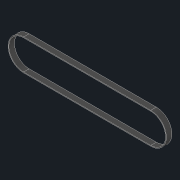
# Autodesk Inventor part: belt4
Saved by Autodesk Inventor 2021 (Build 250183000, 183)
## iProperties
Created: 2021-08-06
Part Number: belt4
Material: ゴム
Document SubType Name: Modeling
Designer: yuta0
Density: 0.93 g/cm^3
Appearance: ゴム - 黒
Author: yuta0
Autodesk Inventor part; units mm, degrees
ref_plane "YZ Plane" through (0, 0, 0) normal (1, 0, 0) x (0, 1, 0)
ref_plane "XZ Plane" through (0, 0, 0) normal (0, 1, 0) x (-1, 0, 0)
ref_plane "XY Plane" through (0, 0, 0) normal (0, 0, 1) x (1, 0, 0)
sketch "スケッチ1" plane through (0, 0, 0) normal (0, 0, 1) x (1, 0, 0)
  line L0 (-68, 0) -> (68, 0) construction
  line L1 (-68, -16.2338) -> (68, -16.2338)
  line L2 (68, 16.2338) -> (-68, 16.2338)
  arc A0 (-68, 16.2338) -> (-68, -16.2338) centre (-68, 0) ccw
  arc A1 (68, -16.2338) -> (68, 16.2338) centre (68, 0) ccw
  line L3 (-68, -16.6528) -> (68, -16.6528)
  arc A2 (68, -16.6528) -> (68, 16.6528) centre (68, 0) ccw
  line L4 (68, 16.6528) -> (-68, 16.6528)
  arc A3 (-68, 16.6528) -> (-68, -16.6528) centre (-68, 0) ccw
  line L5 (-68, -15.8528) -> (68, -15.8528)
  arc A4 (68, -15.8528) -> (68, 15.8528) centre (68, 0) ccw
  line L6 (68, 15.8528) -> (-68, 15.8528)
  arc A5 (-68, 15.8528) -> (-68, -15.8528) centre (-68, 0) ccw
  point P0 (0, 0)
  dimension "d0" = 136
  dimension "d1" = 16.2338
  dimension "d2" = 0.419
  dimension "d3" = 0.8
  constraints: 16 end point, 12 point on circle, 6 centre point, 4 tangent, 3 parallel, 1 horizontal, 1 midpoint, 6 other
  measures "d0" distance of L2.start L2.end
  measures "d1" radius of A0
  measures "d2" radial gap between concentric circles of A0 A3
  measures "d3" radial gap between concentric circles of A3 A5
extrude "押し出し1" add sketch "スケッチ1" along normal mid plane 6 contours A0 L2 A1 L1 | A3 L4 A2 L3
